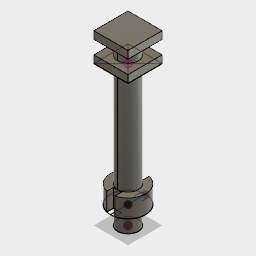
attache ponceuse v1 (Autodesk Fusion 360 design; units mm, degrees)
Autodesk Fusion 360 part; units mm, degrees
note: some values were not read from the file. Set by a fixed rule: which sketch regions a step uses.
sketch "Sketch1" plane through (0, 0, 0) normal (0, 1, 0) x (1, 0, 0)
  circle A0 centre (0, 0) radius 2.875
  dimension "d1" = 5.75
  measures "d1" diameter of A0
extrude "Extrude1" add sketch "Sketch1" along normal blind 5
sketch "Sketch2" plane through (0, 5, 0) normal (0, 1, 0) x (-1, 0, 0)
  circle A0 centre (0, 0) radius 2.875
  circle A1 centre (0, 0) radius 4.875
  line L0 (0, 0) -> (0, 4.875)
  line L1 (1.125, 2.875) -> (-1.125, 2.875)
  line L2 (1.125, 2.875) -> (0, 2.875)
  line L3 (1.125, 2.875) -> (1.125, 4.7434)
  line L4 (-1.125, 2.875) -> (-1.125, 4.7434)
  arc A2 (1.125, 4.7434) -> (-1.125, 4.7434) centre (0, 0) ccw
  line L5 (0, 0) -> (0, -4.875)
  line L6 (-1.125, -2.875) -> (1.125, -2.875)
  line L7 (-1.125, -2.875) -> (0, -2.875)
  line L8 (1.125, -2.875) -> (1.125, -4.7434)
  line L9 (-1.125, -2.875) -> (-1.125, -4.7434)
  dimension "d4" = 9.75
  dimension "d5" = 2.25
  dimension "d9" = 2.25
  measures "d4" diameter of A1
  measures "d5" distance of L1.start L1.end
  measures "d9" distance of L6.start L6.end
extrude "Extrude2" add sketch "Sketch2" along normal blind 5 contours A0 L0 L5 | A0 A1 L1 L2 L3 L6 L8 | A0 L0 L5 | A0 A1 L1 L4 L6 L7 L9 | A1 L5 L6 L8 | A1 L5 L6 L7 L9
extrude "Extrude3" cut sketch "Sketch2" along normal through all contours A1 L0 L1 L4 A2 | A1 L0 L1 L2 L3 A2 | A1 L5 L6 L8 | A1 L5 L6 L7 L9
sketch "Sketch3" plane through (0, 10, 0) normal (0, 1, 0) x (-1, 0, 0)
  line L0 (1.125, -2.875) -> (1.125, -4.7434)
  arc A0 (1.125, -4.7434) -> (1.125, 4.7434) centre (0, 0) ccw
  line L1 (1.125, 4.7434) -> (1.125, 2.875)
  line L2 (1.125, 2.875) -> (-1.125, 2.875)
  line L3 (-1.125, 2.875) -> (-1.125, 4.7434)
  arc A1 (-1.125, 4.7434) -> (-1.125, -4.7434) centre (0, 0) ccw
  line L4 (-1.125, -4.7434) -> (-1.125, -2.875)
  line L5 (-1.125, -2.875) -> (1.125, -2.875)
  circle A2 centre (0, 0) radius 2.875
  point P0 (0, -2.875)
extrude "Extrude4" add sketch "Sketch3" along normal blind 28.8 contours A2
sketch "Sketch4" plane through (0, 38.8, 0) normal (0, 1, 0) x (-1, 0, 0)
  arc A0 (-0.0105, 2.875) -> (0.0105, 2.875) centre (0, 0) ccw
  line L0 (0.0105, 2.875) -> (-0.0105, 2.875)
  line L1 (4.75, 4.75) -> (-4.75, 4.75)
  line L2 (-4.75, 4.75) -> (-4.75, -4.75)
  line L3 (-4.75, -4.75) -> (4.75, -4.75)
  line L4 (4.75, -4.75) -> (4.75, 4.75)
  line L5 (4.75, 4.75) -> (-4.75, -4.75)
  line L6 (4.75, -4.75) -> (-4.75, 4.75)
  dimension "d13" = 9.5
  dimension "d14" = 9.5
  measures "d13" distance of L1.start L3.end
  measures "d14" distance of L1.start L1.end
extrude "Extrude5" add sketch "Sketch4" along normal blind 7.9 contours A0 L0 L5 L6 | A0 L5 L6 | A0 L5 L6 | A0 L5 L6
extrude "Extrude6" add sketch "Sketch4" along normal blind 2.1 contours A0 L0 L1 L5 L6 | A0 L2 L5 L6 | A0 L3 L5 L6 | A0 L4 L5 L6
sketch "Sketch5" plane through (0, 46.7, 0) normal (0, 1, 0) x (-1, 0, 0)
  line L0 (0.0105, 2.875) -> (-0.0105, 2.875)
  arc A0 (-0.0105, 2.875) -> (0.0105, 2.875) centre (0, 0) ccw
  line L1 (4.75, 4.75) -> (-4.75, 4.75)
  line L2 (-4.75, 4.75) -> (-4.75, -4.75)
  line L3 (-4.75, -4.75) -> (4.75, -4.75)
  line L4 (4.75, -4.75) -> (4.75, 4.75)
  point P0 (4.75, 4.75)
  point P1 (-4.75, -4.75)
extrude "Extrude7" add sketch "Sketch5" against normal blind 2.1
